Barrel Mount End Cap_v2 (Autodesk Fusion 360 design; units mm, degrees)
Autodesk Fusion 360 part; units mm, degrees
sketch "Sketch1" plane through (0, 0, 0) normal (0, 1, 0) x (1, 0, 0)
  arc A0 (8.5414, -3.1214) -> (8.2, -3.2628) centre (8.4, -3.2628) ccw
  arc A1 (-3.1214, -8.5414) -> (-3.2628, -8.2) centre (-3.2628, -8.4) ccw
  line L0 (-3.1214, 8.5414) -> (-4.4312, 9.8494)
  line L1 (4.4022, 9.8222) -> (3.1214, 8.5414)
  arc A2 (-8.5414, 3.1214) -> (-8.2, 3.2628) centre (-8.4, 3.2628) ccw
  line L2 (-10, 9.5) -> (-10.0001, 4.8314)
  line L3 (-5.5, 6.5607) -> (-5.5, 8.2)
  line L4 (-9.8494, 4.4312) -> (-8.5414, 3.1214)
  line L5 (3.9, 2.8393) -> (6.5607, 5.5)
  arc A3 (-10.0001, 4.8314) -> (-9.8494, 4.4312) centre (-9.372, 4.8395) ccw
  arc A4 (3.1214, 8.5414) -> (3.2628, 8.2) centre (3.2628, 8.4) ccw
  arc A5 (-3.2628, 8.2) -> (-3.1214, 8.5414) centre (-3.2628, 8.4) ccw
  line L6 (-2.8393, -3.9) -> (2.8393, -3.9)
  circle A6 centre (0, 0) radius 2.1
  arc A7 (-4.4312, 9.8494) -> (-4.8314, 10) centre (-4.8314, 9.3929) ccw
  line L7 (6.5607, 5.5) -> (8.2, 5.5)
  line L8 (10, 4.8314) -> (10, 9.5)
  line L9 (-2.8393, 3.9) -> (-5.5, 6.5607)
  line L10 (9.5, 10) -> (4.8314, 10)
  line L11 (-8.2, 3.2628) -> (-8.2, 5.5)
  line L12 (10, -9.5) -> (10, -4.8314)
  line L13 (5.5, 6.5607) -> (2.8393, 3.9)
  line L14 (-3.9, -2.8393) -> (-6.5607, -5.5)
  line L15 (3.2628, 8.2) -> (5.5, 8.2)
  line L16 (-5.5, 8.2) -> (-3.2628, 8.2)
  arc A8 (-4.8314, -10) -> (-4.4022, -9.8222) centre (-4.8314, -9.3929) ccw
  line L17 (9.8222, -4.4022) -> (8.5414, -3.1214)
  line L18 (-3.2628, -8.2) -> (-5.5, -8.2)
  line L19 (6.5607, -5.5) -> (3.9, -2.8393)
  arc A9 (-9.8222, -4.4022) -> (-9.9987, -4.7917) centre (-9.3929, -4.8314) ccw
  arc A10 (9.5, -10) -> (10, -9.5) centre (9.5, -9.5) ccw
  line L20 (-8.5414, -3.1214) -> (-9.8222, -4.4022)
  arc A11 (-10, -9.5) -> (-9.5, -10) centre (-9.5, -9.5) ccw
  arc A12 (10, -4.8314) -> (9.8222, -4.4022) centre (9.3929, -4.8314) ccw
  line L21 (-4.8314, 10) -> (-9.5, 10)
  line L22 (-8.2, 5.5) -> (-6.5607, 5.5)
  line L23 (3.9, -2.8393) -> (3.9, 2.8393)
  line L24 (-3.9, 2.8393) -> (-3.9, -2.8393)
  arc A13 (-9.5, 10) -> (-10, 9.5) centre (-9.5, 9.5) ccw
  arc A14 (8.2, 3.2628) -> (8.5414, 3.1214) centre (8.4, 3.2628) ccw
  arc A15 (4.8314, 10) -> (4.4022, 9.8222) centre (4.8314, 9.3929) ccw
  line L25 (5.5, 8.2) -> (5.5, 6.5607)
  arc A16 (10, 9.5) -> (9.5, 10) centre (9.5, 9.5) ccw
  arc A17 (9.8222, 4.4022) -> (10, 4.8314) centre (9.3929, 4.8314) ccw
  line L26 (-6.5607, 5.5) -> (-3.9, 2.8393)
  line L27 (2.8393, -3.9) -> (5.5, -6.5607)
  line L28 (-5.5, -8.2) -> (-5.5, -6.5607)
  line L29 (-4.4022, -9.8222) -> (-3.1214, -8.5414)
  arc A18 (4.2336, -9.6536) -> (4.8314, -10) centre (4.8837, -9.2207) ccw
  arc A19 (3.2628, -8.2) -> (3.1214, -8.5414) centre (3.2628, -8.4) ccw
  line L30 (-8.2, -5.5) -> (-8.2, -3.2628)
  line L31 (3.1214, -8.5414) -> (4.2336, -9.6536)
  line L32 (8.2, -5.5) -> (6.5607, -5.5)
  line L33 (-5.5, -6.5607) -> (-2.8393, -3.9)
  line L34 (-6.5607, -5.5) -> (-8.2, -5.5)
  line L35 (5.5, -6.5607) -> (5.5, -8.2)
  line L36 (8.2, -3.2628) -> (8.2, -5.5)
  line L37 (5.5, -8.2) -> (3.2628, -8.2)
  line L38 (-9.9987, -4.7917) -> (-10, -9.5)
  line L39 (-9.5, -10) -> (-4.8314, -10)
  line L40 (4.8314, -10) -> (9.5, -10)
  arc A20 (-8.2, -3.2628) -> (-8.5414, -3.1214) centre (-8.4, -3.2628) ccw
  line L41 (8.5414, 3.1214) -> (9.8222, 4.4022)
  line L42 (8.2, 5.5) -> (8.2, 3.2628)
  line L43 (2.8393, 3.9) -> (-2.8393, 3.9)
  line L44 (-10.0001, -10) -> (10, -10)
  line L45 (10, -10) -> (10, 10)
  line L46 (10, 10) -> (-10.0001, 10)
  line L47 (-10.0001, 10) -> (-10.0001, -10)
  line L48 (2.7979, -4) -> (5.4, -6.6021)
  line L49 (5.4, -6.6021) -> (5.4, -8.1)
  line L50 (5.4, -8.1) -> (3.2628, -8.1)
  arc A21 (3.2628, -8.1) -> (3.0507, -8.6121) centre (3.2628, -8.4) ccw
  line L51 (3.0507, -8.6121) -> (4.1561, -9.7175)
  arc A22 (4.1561, -9.7175) -> (4.8282, -10.1) centre (4.8837, -9.2207) ccw
  line L52 (4.8282, -10.1) -> (9.5, -10.1)
  arc A23 (9.5, -10.1) -> (10.1, -9.5) centre (9.5, -9.5) ccw
  line L53 (10.1, -9.5) -> (10.1, -4.8314)
  arc A24 (10.1, -4.8314) -> (9.8929, -4.3315) centre (9.3929, -4.8314) ccw
  line L54 (9.8929, -4.3315) -> (8.6121, -3.0507)
  arc A25 (8.6121, -3.0507) -> (8.1, -3.2628) centre (8.4, -3.2628) ccw
  line L55 (8.1, -3.2628) -> (8.1, -5.4)
  line L56 (8.1, -5.4) -> (6.6021, -5.4)
  line L57 (6.6021, -5.4) -> (4, -2.7979)
  line L58 (4, -2.7979) -> (4, 2.7979)
  line L59 (4, 2.7979) -> (6.6021, 5.4)
  line L60 (6.6021, 5.4) -> (8.1, 5.4)
  line L61 (8.1, 5.4) -> (8.1, 3.2628)
  arc A26 (8.1, 3.2628) -> (8.6121, 3.0507) centre (8.4, 3.2628) ccw
  line L62 (8.6121, 3.0507) -> (9.8929, 4.3315)
  arc A27 (9.8929, 4.3315) -> (10.1, 4.8314) centre (9.3929, 4.8314) ccw
  line L63 (10.1, 4.8314) -> (10.1, 9.5)
  arc A28 (10.1, 9.5) -> (9.5, 10.1) centre (9.5, 9.5) ccw
  line L64 (9.5, 10.1) -> (4.8314, 10.1)
  arc A29 (4.8314, 10.1) -> (4.3315, 9.8929) centre (4.8314, 9.3929) ccw
  line L65 (4.3315, 9.8929) -> (3.0507, 8.6121)
  arc A30 (3.0507, 8.6121) -> (3.2628, 8.1) centre (3.2628, 8.4) ccw
  line L66 (3.2628, 8.1) -> (5.4, 8.1)
  line L67 (5.4, 8.1) -> (5.4, 6.6021)
  line L68 (5.4, 6.6021) -> (2.7979, 4)
  line L69 (2.7979, 4) -> (-2.7979, 4)
  line L70 (-2.7979, 4) -> (-5.4, 6.6021)
  line L71 (-5.4, 6.6021) -> (-5.4, 8.1)
  line L72 (-5.4, 8.1) -> (-3.2628, 8.1)
  arc A31 (-3.2628, 8.1) -> (-3.0509, 8.6124) centre (-3.2628, 8.4) ccw
  line L73 (-3.0509, 8.6124) -> (-4.3627, 9.9223)
  arc A32 (-4.3627, 9.9223) -> (-4.8314, 10.1) centre (-4.8314, 9.3929) ccw
  line L74 (-4.8314, 10.1) -> (-9.5, 10.1)
  arc A33 (-9.5, 10.1) -> (-10.1, 9.5) centre (-9.5, 9.5) ccw
  line L75 (-10.1, 9.5) -> (-10.1001, 4.8308)
  arc A34 (-10.1001, 4.8308) -> (-9.9227, 4.3632) centre (-9.372, 4.8395) ccw
  line L76 (-9.9227, 4.3632) -> (-8.6124, 3.0509)
  arc A35 (-8.6124, 3.0509) -> (-8.1, 3.2628) centre (-8.4, 3.2628) ccw
  line L77 (-8.1, 3.2628) -> (-8.1, 5.4)
  line L78 (-8.1, 5.4) -> (-6.6021, 5.4)
  line L79 (-6.6021, 5.4) -> (-4, 2.7979)
  line L80 (-4, 2.7979) -> (-4, -2.7979)
  line L81 (-4, -2.7979) -> (-6.6021, -5.4)
  line L82 (-6.6021, -5.4) -> (-8.1, -5.4)
  line L83 (-8.1, -5.4) -> (-8.1, -3.2628)
  arc A36 (-8.1, -3.2628) -> (-8.6121, -3.0507) centre (-8.4, -3.2628) ccw
  line L84 (-8.6121, -3.0507) -> (-9.8929, -4.3315)
  arc A37 (-9.8929, -4.3315) -> (-10.0987, -4.7886) centre (-9.3929, -4.8314) ccw
  line L85 (-10.0987, -4.7886) -> (-10.1, -9.4997)
  arc A38 (-10.1, -9.4997) -> (-9.5, -10.1) centre (-9.5, -9.5) ccw
  line L86 (-9.5, -10.1) -> (-4.8314, -10.1)
  arc A39 (-4.8314, -10.1) -> (-4.3315, -9.8929) centre (-4.8314, -9.3929) ccw
  line L87 (-4.3315, -9.8929) -> (-3.0507, -8.6121)
  arc A40 (-3.0507, -8.6121) -> (-3.2628, -8.1) centre (-3.2628, -8.4) ccw
  line L88 (-3.2628, -8.1) -> (-5.4, -8.1)
  line L89 (-5.4, -8.1) -> (-5.4, -6.6021)
  line L90 (-5.4, -6.6021) -> (-2.7979, -4)
  line L91 (-2.7979, -4) -> (2.7979, -4)
  line L92 (10, 4.8314) -> (-10.0001, 4.8314) construction
  line L93 (-10.0001, -9.5201) -> (-9.9995, -9.5226)
  constraint horizontal L44
  constraint vertical L45
  constraint horizontal L46
  constraint vertical L47
  constraint coincident L47 L2.end
  constraint perpendicular L45 L92
  constraint parallel L27 L48
  constraint parallel L35 L49
  constraint parallel L37 L50
  constraint concentric A19 A21
  constraint parallel L31 L51
  constraint concentric A18 A22
  constraint parallel L40 L52
  constraint concentric A10 A23
  constraint parallel L12 L53
  constraint concentric A12 A24
  constraint parallel L17 L54
  constraint concentric A0 A25
  constraint parallel L36 L55
  constraint parallel L32 L56
  constraint parallel L19 L57
  constraint parallel L23 L58
  constraint parallel L5 L59
  constraint parallel L7 L60
  constraint parallel L42 L61
  constraint concentric A14 A26
  constraint parallel L41 L62
  constraint concentric A17 A27
  constraint parallel L8 L63
  constraint concentric A16 A28
  constraint parallel L10 L64
  constraint concentric A15 A29
  constraint parallel L1 L65
  constraint concentric A4 A30
  constraint parallel L15 L66
  constraint parallel L25 L67
  constraint parallel L13 L68
  constraint parallel L43 L69
  constraint parallel L9 L70
  constraint parallel L3 L71
  constraint parallel L16 L72
  constraint concentric A5 A31
  constraint parallel L0 L73
  constraint concentric A7 A32
  constraint parallel L21 L74
  constraint concentric A13 A33
  constraint parallel L2 L75
  constraint concentric A3 A34
  constraint parallel L4 L76
  constraint concentric A2 A35
  constraint parallel L11 L77
  constraint parallel L22 L78
  constraint parallel L26 L79
  constraint parallel L24 L80
  constraint parallel L14 L81
  constraint parallel L34 L82
  constraint parallel L30 L83
  constraint concentric A20 A36
  constraint parallel L20 L84
  constraint concentric A9 A37
  constraint parallel L38 L85
  constraint concentric A11 A38
  constraint parallel L39 L86
  constraint concentric A8 A39
  constraint parallel L29 L87
  constraint concentric A1 A40
  constraint parallel L18 L88
  constraint parallel L28 L89
  constraint parallel L33 L90
  constraint parallel L6 L91
  constraint tangent A21 L51
  constraint tangent A26 L62
  constraint tangent L50 A21
  constraint tangent L65 A30
  constraint tangent L54 A25
  constraint tangent A36 L84
  constraint tangent A25 L55
  constraint tangent L72 A31
  constraint tangent L61 A26
  constraint tangent A40 L88
  constraint tangent A30 L66
  constraint tangent A35 L77
  constraint tangent L87 A40
  constraint tangent L83 A36
  constraint coincident L47 L93.start
  constraint coincident A11 L93.end
extrude "Extrude2" add sketch "Sketch1" against normal blind 4 contours A0 A1 L0 L1 A2 L2 L3 L4 L5 A3 A4 A5 L6 A7 L7 L8 L9 L10 L11 L12 L13 L14 L15 L16 A8 L17 L18 L19 A9 A10 L20 A11 A12 L21 L22 L23 L24 A13 A14 A15 L25 A16 A17 L26 L27 L28 L29 A18 A19 L30 L31 L32 L33 L34 L35 L36 L37 L38 L39 L40 A20 L41 L42 L43 L44 L45 L46 L47 | A0 L5 L7 L17 L19 A12 L23 A14 A17 L32 L36 L41 L42 L45 A24 L54 A25 L55 L56 L57 L58 L59 L60 L61 A26 L62 A27 | A10 L44 L45 A23 | L45 A24 L54 A25 L55 L56 L57 L58 L59 L60 L61 A26 L62 A27 | L44 L45 A23 | A1 L6 A8 L18 L27 L28 L29 A18 A19 L31 L33 L35 L37 L44 L48 L49 L50 A21 L51 A22 A39 L87 A40 L88 L89 L90 L91 | L44 L48 L49 L50 A21 L51 A22 A39 L87 A40 L88 L89 L90 L91 | A16 L45 L46 A28 | L45 L46 A28 | L0 L1 L3 A4 A5 A7 L9 L13 L15 L16 A15 L25 L43 L46 A29 L65 A30 L66 L67 L68 L69 L70 L71 L72 A31 L73 A32 | L46 A29 L65 A30 L66 L67 L68 L69 L70 L71 L72 A31 L73 A32 | A2 L4 A3 L11 L14 A9 L20 L22 L24 L26 L30 L34 A20 L47 A34 L76 A35 L77 L78 L79 L80 L81 L82 L83 A36 L84 A37 | L47 A34 L76 A35 L77 L78 L79 L80 L81 L82 L83 A36 L84 A37 | A6
extrude "Extrude3" add sketch "Sketch1" along normal blind 3 contours L45 A24 L54 A25 L55 L56 L57 L58 L59 L60 L61 A26 L62 A27 | L44 L48 L49 L50 A21 L51 A22 A39 L87 A40 L88 L89 L90 L91 | L46 A29 L65 A30 L66 L67 L68 L69 L70 L71 L72 A31 L73 A32 | L47 A34 L76 A35 L77 L78 L79 L80 L81 L82 L83 A36 L84 A37
chamfer "Chamfer1" distance 2 angle 45 4 edges at (0.25, -4, 10) (-10.0001, -4, 2.3443) (-10.0001, -4, -7.1657) (0.25, -4, -10) tangent chain off
